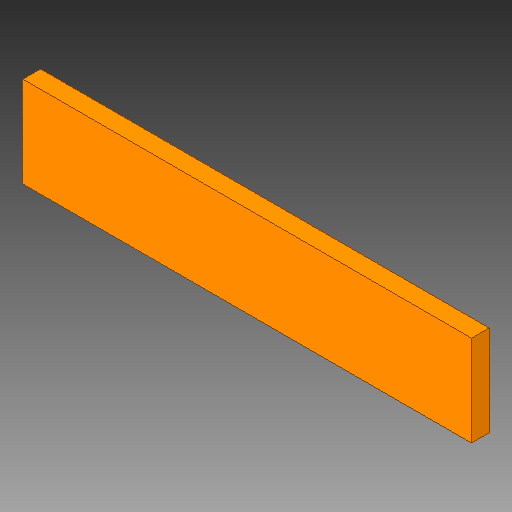
# Autodesk Inventor part: 2X10
Saved by Autodesk Inventor 2018 (Build 220112000, 112)
## iProperties
Created: 2015-11-24
Part Number: 2X10
Material: Generic
Document SubType Name: Modeling
Designer: PhillipD
Density: 1 g/cm^3
Appearance: 2X10, 2X10
Author: PhillipD
Autodesk Inventor part; units mm, degrees
ref_plane "YZ Plane" through (0, 0, 0) normal (1, 0, 0) x (0, 1, 0)
ref_plane "XZ Plane" through (0, 0, 0) normal (0, 1, 0) x (-1, 0, 0)
ref_plane "XY Plane" through (0, 0, 0) normal (0, 0, 1) x (1, 0, 0)
sketch "2X10, 2X10_51" plane through (0, 0, 0) normal (0, 0, 1) x (1, 0, 0)
  line L0 (-12.7762, 2.54) -> (12.7, 2.54)
  line L1 (12.7, 2.54) -> (12.7, -2.6162)
  line L2 (12.7, -2.6162) -> (-12.7762, -2.6162)
  line L3 (-12.7762, -2.6162) -> (-12.7762, 2.54)
  constraints: 8 end point
extrude "Extrusion1" add sketch "2X10, 2X10_51" along normal blind 1
body "Solid1"
